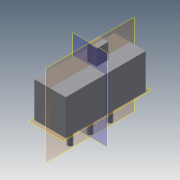
# Autodesk Inventor part: SS-12SDP2
Saved by Autodesk Inventor 2015 SP1 (Build 190203100, 203)
## iProperties
Created: 2015-04-14
Part Number: SS-12SDP2
Material: 一般
Document SubType Name: Modeling
Designer: Yamaura
Density: 1 g/cm^3
Appearance: 既定
Author: Yamaura
Autodesk Inventor part; units mm, degrees
sketch "スケッチ1" plane through (0, 0, 0) normal (0, 0, 1) x (1, 0, 0)
  line L0 (-2, 5.1) -> (2, 5.1)
  line L1 (2, 5.1) -> (2, -5.1)
  line L2 (2, -5.1) -> (-2, -5.1)
  line L3 (-2, -5.1) -> (-2, 5.1)
  point P0 (0, 0)
  dimension "d0" = 2
  dimension "d1" = 4
  dimension "d2" = 5.1
  dimension "d3" = 10.2
  constraints: 8 end point, 2 parallel, 1 horizontal, 1 perpendicular
  measures "d0" distance from line of L3 point (0, 0)
  measures "d1" distance of L0.start L0.end
  measures "d2" distance from line of L0 point (0, 0)
  measures "d3" distance of L2.end L0.start
extrude "押し出し1" add sketch "スケッチ1" along normal blind 4.5
sketch "スケッチ4" plane through (0, 0, 0) normal (0, 0, 1) x (1, 0, 0)
  circle A0 centre (0, 2.54) radius 0.3
  circle A1 centre (0, 0) radius 0.3
  circle A2 centre (0, -2.54) radius 0.3
  dimension "d16" = 0.6
  dimension "d17" = 0.6
  dimension "d18" = 0.6
  dimension "d19" = 2.54
  dimension "d20" = 2.54
  constraints: 3 centre point, 1 coincident
  measures "d16" diameter of A0
  measures "d17" diameter of A1
  measures "d18" diameter of A2
  measures "d19" distance of point (0, 0) A0.centre
  measures "d20" distance of point (0, 0) A2.centre
extrude "押し出し3" add sketch "スケッチ4" against normal blind 3
sketch "スケッチ5" plane through (0, 0, 0) normal (0, 0, 1) x (1, 0, 0)
  line L0 (-0.6, 1.75) -> (0.6, 1.75)
  line L1 (0.6, 1.75) -> (0.6, 0.25)
  line L2 (0.6, 0.25) -> (-0.6, 0.25)
  line L3 (-0.6, 0.25) -> (-0.6, 1.75)
  line L4 (0.6, 0.25) -> (-0.6, 1.75)
  line L5 (0.6, 1.75) -> (-0.6, 0.25)
  line L6 (0, -0.35) -> (0, 2.1) projected
  line L7 (-0.84, 0) -> (0.84, 0) projected
  point P0 (0, 0)
  point P1 (0, 1)
  point P2 (0, 1)
  dimension "d23" = 1
  dimension "d24" = 1.5
  dimension "d25" = 1.2
  constraints: 12 end point, 3 midpoint, 2 parallel, 1 horizontal, 1 perpendicular, 1 point on line
  measures "d23" distance from line of L7 point (0, 1)
  measures "d24" distance of L2.end L0.start
  measures "d25" distance of L0.start L0.end
extrude "押し出し4" add sketch "スケッチ5" along normal blind 6.5
